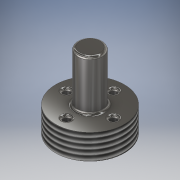
# Autodesk Inventor part: Disco2
Saved by Autodesk Inventor 2019 (Build 230136000, 136)
## iProperties
Created: 2021-12-02
Part Number: Disco2
Material: Generic
Document SubType Name: Modeling
Designer: Alex
Density: 1 g/cm^3
Appearance: Steel - Polished
Author: Alex
Autodesk Inventor part; units mm, degrees
ref_plane "YZ Plane" through (0, 0, 0) normal (1, 0, 0) x (0, 1, 0)
ref_plane "XZ Plane" through (0, 0, 0) normal (0, 1, 0) x (-1, 0, 0)
ref_plane "XY Plane" through (0, 0, 0) normal (0, 0, 1) x (1, 0, 0)
sketch "Sketch3" plane through (0, 0, 0) normal (0, 1, 0) x (-1, 0, 0)
  circle A0 centre (0, 0) radius 27.5
  circle A1 centre (18.75, 0) radius 2.5
  circle A2 centre (0, -18.75) radius 2.5
  circle A3 centre (-18.75, 0) radius 2.5
  circle A4 centre (0, 18.75) radius 2.5
  dimension "d15" = 55
  dimension "d17" = 5
  dimension "d18" = 5
  dimension "d19" = 5
  dimension "d20" = 5
  constraints: 5 centre point, 1 coincident
  measures "d15" diameter of A0
  measures "d17" diameter of A1
  measures "d18" diameter of A2
  measures "d19" diameter of A3
  measures "d20" diameter of A4
extrude "Extrusion3" add sketch "Sketch3" along normal blind 20
sketch "Sketch4" plane through (0, 20, 0) normal (0, 1, 0) x (1, 0, 0)
  circle A0 centre (0, 0) radius 10
  dimension "d23" = 20
  constraints: 1 centre point, 1 coincident
  measures "d23" diameter of A0
extrude "Extrusion4" add sketch "Sketch4" along normal blind 40
fillet "Fillet5" radius 2 6 edges at (-10, 60, 0) (21.25, 20, 0) (2.5, 20, -18.75) (-16.25, 20, 0) (2.5, 20, 18.75) (-10, 20, 0)
thread "Thread2" size "M55x4" class "6g" standard "ANSI Metric M Profile" full length
body "Solid2"
